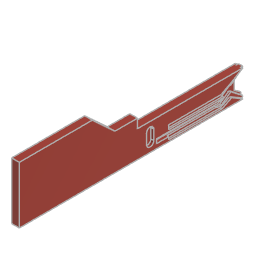
4ks (Autodesk Fusion 360 design; units mm, degrees)
Autodesk Fusion 360 part; units mm, degrees
note: some values were not read from the file. Set by a fixed rule: which face or edge a step refers to.
sketch "blade" plane through (0, 0, 0) normal (1, 0, 0) x (0, 1, 0)
  line L0 (0, 0) -> (0, 0.75) construction
  line L1 (0, 0.75) -> (25.25, 0.75)
  line L2 (25.25, 0.75) -> (25.25, 8.75)
  line L3 (25.25, 8.75) -> (0, 8.75)
  line L4 (0, 8.75) -> (0, 0.75)
  dimension "d13" = 0.75
  dimension "d14" = 25.25
  dimension "d15" = 8
  constraint coincident L0.start origin
  constraint vertical L0
  constraint horizontal L1
  constraint vertical L2
  constraint horizontal L3
  constraint vertical L4
  measures "d13" distance of L0.start L0.end
  measures "d14" distance of L0.end L1.end
  measures "d15" distance of L0.end L3.end
extrude "Extrude1" add sketch "blade" along normal blind 1.1 makes body 1
sketch "single track" plane through (1.1, 0, 0) normal (1, 0, 0) x (0, 1, 0)
  line L0 (0, 8.75) -> (0, 0.75)
  line L1 (0, 0.75) -> (25.25, 0.75)
  line L2 (25.25, 0.75) -> (25.25, 8.75)
  line L3 (25.25, 8.75) -> (0, 8.75)
  line L4 (0, 0.75) -> (0.9, 0.75) construction
  line L5 (0.9, 0.75) -> (4.4, 0.75) construction
  line L6 (4.4, 0.75) -> (7.9, 0.75) construction
  line L7 (7.9, 0.75) -> (11.4, 0.75) construction
  line L8 (11.4, 0.75) -> (14.9, 0.75) construction
  line L9 (14.9, 0.75) -> (18.4, 0.75) construction
  line L10 (18.4, 0.75) -> (21.9, 0.75) construction
  line L11 (21.9, 0.75) -> (21.9, 4.75) construction
  line L12 (21.9, 4.75) -> (25.25, 4.75)
  line L13 (0.9, 0.75) -> (0.9, 2.75) construction
  line L14 (4.4, 0.75) -> (4.4, 2.75) construction
  line L15 (7.9, 0.75) -> (7.9, 2.75) construction
  line L16 (11.4, 0.75) -> (11.4, 2.75) construction
  line L17 (14.9, 0.75) -> (14.9, 2.75) construction
  line L18 (18.4, 0.75) -> (18.4, 2.75) construction
  circle A0 centre (0.9, 2.75) radius 0.6 construction
  circle A1 centre (4.4, 2.75) radius 0.6 construction
  circle A2 centre (7.9, 2.75) radius 0.6 construction
  circle A3 centre (11.4, 2.75) radius 0.6 construction
  circle A4 centre (14.9, 2.75) radius 0.6 construction
  circle A5 centre (18.4, 2.75) radius 0.85 construction
  line L19 (0.9, 2.75) -> (0, 2.75)
  line L20 (0, 0.75) -> (0, 2.75) construction
  line L21 (0.9, 2.75) -> (1.2, 2.75)
  line L22 (4.4, 2.75) -> (4.1, 2.75)
  line L23 (4.4, 2.75) -> (4.7, 2.75)
  line L24 (7.9, 2.75) -> (7.6, 2.75)
  line L25 (7.9, 2.75) -> (8.2, 2.75)
  line L26 (11.4, 2.75) -> (11.1, 2.75)
  line L27 (11.4, 2.75) -> (11.7, 2.75)
  line L28 (14.9, 2.75) -> (14.6, 2.75)
  line L29 (14.9, 2.75) -> (15.2, 2.75)
  line L30 (18.4, 2.75) -> (18.1, 2.75)
  line L31 (18.4, 2.75) -> (18.7, 2.75)
  line L32 (21.9, 4.75) -> (21.6, 4.75)
  line L33 (1.2, 2.75) -> (4.1, 2.75)
  line L34 (4.7, 2.75) -> (7.6, 2.75)
  line L35 (8.2, 2.75) -> (11.1, 2.75)
  line L36 (11.7, 2.75) -> (14.6, 2.75)
  line L37 (15.2, 2.75) -> (18.1, 2.75)
  line L38 (18.7, 2.75) -> (21.6, 4.75)
  dimension "d18" = 0.9
  dimension "d19" = 3.5
  dimension "d20" = 3.5
  dimension "d21" = 3.5
  dimension "d22" = 3.5
  dimension "d23" = 3.5
  dimension "d24" = 3.5
  dimension "d25" = 2
  dimension "d26" = 2
  dimension "d27" = 2
  dimension "d28" = 2
  dimension "d29" = 2
  dimension "d30" = 2
  dimension "d31" = 1.2
  dimension "d32" = 1.2
  dimension "d33" = 1.2
  dimension "d34" = 1.2
  dimension "d35" = 1.2
  dimension "d36" = 1.7
  dimension "d37" = 0.3
  dimension "d38" = 0.3
  dimension "d39" = 0.3
  dimension "d40" = 0.3
  dimension "d41" = 0.3
  dimension "d42" = 0.3
  dimension "d43" = 0.3
  dimension "d44" = 0.3
  dimension "d45" = 0.3
  dimension "d46" = 0.3
  dimension "d47" = 0.3
  dimension "d48" = 0.3
  constraint coincident L0.end L1.start
  constraint coincident L1 L4.end
  constraint parallel L1 L5
  constraint parallel L1 L6
  constraint parallel L1 L7
  constraint parallel L1 L8
  constraint parallel L1 L9
  constraint parallel L1 L10
  constraint perpendicular L10 L11
  constraint midpoint L2 L12.end
  constraint perpendicular L2 L12
  constraint perpendicular L4 L13
  constraint perpendicular L5 L14
  constraint perpendicular L6 L15
  constraint perpendicular L8 L16
  constraint perpendicular L9 L17
  constraint perpendicular L10 L18
  constraint coincident L13.end A0.centre
  constraint coincident L14.end A1.centre
  constraint coincident L15.end A2.centre
  constraint coincident L16.end A3.centre
  constraint coincident L17.end A4.centre
  constraint coincident L18.end A5.centre
  constraint coincident L0 L19.end
  constraint perpendicular L0 L19
  constraint perpendicular L13 L21
  constraint perpendicular L14 L22
  constraint perpendicular L14 L23
  constraint perpendicular L15 L24
  constraint perpendicular L15 L25
  constraint perpendicular L16 L26
  constraint perpendicular L16 L27
  constraint perpendicular L17 L28
  constraint perpendicular L17 L29
  constraint perpendicular L18 L30
  constraint perpendicular L18 L31
  constraint perpendicular L11 L32
  measures "d18" distance of L0.end L4.end
  measures "d19" distance of L4.end L5.end
  measures "d20" distance of L5.end L6.end
  measures "d21" distance of L6.end L7.end
  measures "d22" distance of L7.end L8.end
  measures "d23" distance of L8.end L9.end
  measures "d24" distance of L9.end L10.end
  measures "d25" distance of L4.end L13.end
  measures "d26" distance of L5.end L14.end
  measures "d27" distance of L6.end L15.end
  measures "d28" distance of L7.end L16.end
  measures "d29" distance of L8.end L17.end
  measures "d30" distance of L9.end L18.end
  measures "d31" diameter of A0
  measures "d32" diameter of A1
  measures "d33" diameter of A2
  measures "d34" diameter of A3
  measures "d35" diameter of A4
  measures "d36" diameter of A5
  measures "d37" distance of L13.end L21.end
  measures "d38" distance of L14.end L22.end
  measures "d39" distance of L14.end L23.end
  measures "d40" distance of L15.end L24.end
  measures "d41" distance of L15.end L25.end
  measures "d42" distance of L16.end L26.end
  measures "d43" distance of L16.end L27.end
  measures "d44" distance of L17.end L28.end
  measures "d45" distance of L17.end L29.end
  measures "d46" distance of L18.end L30.end
  measures "d47" distance of L18.end L31.end
  measures "d48" distance of L11.end L32.end
sketch "single track cutter" plane through (0, 0, 0) normal (0, -1, 0) x (1, 0, 0)
  line L0 (0, 8.75) -> (0, 0.75)
  line L1 (0, 0.75) -> (1.1, 0.75)
  line L2 (1.1, 0.75) -> (1.1, 8.75)
  line L3 (1.1, 8.75) -> (0, 8.75)
  line L4 (1.1, 2.75) -> (1.1, 2.15)
  line L5 (1.1, 2.75) -> (1.1, 3.35)
  line L6 (1.1, 3.35) -> (0.1, 3.35)
  line L7 (0.1, 3.35) -> (0.1, 2.15)
  line L8 (0.1, 2.15) -> (1.1, 2.15)
  point P0 (1.1, 2.75)
  dimension "d49" = 0.6
  dimension "d50" = 0.6
  dimension "d51" = 1
  constraint vertical L4
  constraint coincident P0 L4.start
  constraint parallel L2 L5
  constraint perpendicular L5 L6
  constraint perpendicular L6 L7
  constraint perpendicular L4 L8
  measures "d49" distance of P0 L4.end
  measures "d50" distance of P0 L5.end
  measures "d51" distance of L5.end L6.end
sketch "wider single track" plane through (1.1, 0, 0) normal (1, 0, 0) x (0, 1, 0)
  line L0 (0, 8.75) -> (0, 0.75)
  line L1 (0, 0.75) -> (25.25, 0.75)
  line L2 (25.25, 0.75) -> (25.25, 8.75)
  line L3 (25.25, 8.75) -> (0, 8.75)
  line L4 (0, 0.75) -> (18.4, 0.75) construction
  line L5 (18.4, 0.75) -> (21.9, 0.75) construction
  line L6 (21.9, 0.75) -> (21.9, 4.75) construction
  line L7 (21.9, 4.75) -> (25.25, 4.75)
  line L8 (18.4, 0.75) -> (18.4, 2.75) construction
  line L9 (18.4, 2.75) -> (18.15, 2.5) construction
  line L10 (18.4, 2.75) -> (18.31, 2.75) construction
  line L11 (18.4, 2.75) -> (18.15, 3) construction
  line L12 (18.4, 2.75) -> (18.31, 2.75) construction
  line L13 (18.4, 2.75) -> (18.31, 2.75) construction
  line L14 (18.15, 3) -> (18.15, 3.6) construction
  line L15 (18.15, 2.5) -> (18.15, 1.9) construction
  line L16 (18.4, 2.75) -> (18.6954, 2.75) construction
  arc A0 (18.6954, 2.75) -> (18.15, 3.6) centre (18.15, 3) ccw
  arc A1 (18.15, 1.9) -> (18.6954, 2.75) centre (18.15, 2.5) ccw
  line L17 (18.4, 2.75) -> (17.6046, 2.75) construction
  arc A2 (18.15, 3.6) -> (17.6046, 2.75) centre (18.15, 3) ccw
  arc A3 (17.6046, 2.75) -> (18.15, 1.9) centre (18.15, 2.5) ccw
  line L18 (18.4, 2.75) -> (18.15, 2.75)
  line L19 (18.4, 2.75) -> (18.825, 2.75)
  line L20 (21.9, 4.75) -> (21.6, 4.75)
  line L21 (18.825, 2.75) -> (21.6, 4.75)
  dimension "d52" = 18.4
  dimension "d53" = 3.5
  dimension "d54" = 2
  dimension "d55" = 45
  dimension "d56" = 0.3536
  dimension "d57" = 45
  dimension "d58" = 0.3536
  dimension "d59" = 0.09
  dimension "d60" = 0.6
  dimension "d61" = 0.6
  dimension "d62" = 0.25
  dimension "d63" = 0.425
  dimension "d64" = 0.3
  constraint coincident L0.end L1.start
  constraint perpendicular L0 L4
  constraint parallel L1 L5
  constraint perpendicular L5 L6
  constraint midpoint L2 L7.end
  constraint perpendicular L2 L7
  constraint perpendicular L4 L8
  constraint horizontal L10
  constraint horizontal L12
  constraint perpendicular L8 L13
  constraint vertical L14
  constraint parallel L8 L15
  constraint perpendicular L8 L16
  constraint coincident L16 A0.start
  constraint coincident L11.end L14.start
  constraint coincident L16.end A0.start
  constraint coincident L9 L15.start
  constraint perpendicular L8 L17
  constraint coincident L17 A2.end
  constraint coincident L17.end A2.end
  constraint perpendicular L8 L18
  constraint perpendicular L8 L19
  constraint perpendicular L6 L20
  measures "d52" distance of L0.end L4.end
  measures "d53" distance of L4.end L5.end
  measures "d54" distance of L4.end L8.end
  measures "d55" angle of L9 L10
  measures "d56" distance of L8.end L9.end
  measures "d57" angle of L11 L12
  measures "d58" distance of L8.end L11.end
  measures "d59" distance of L8.end L10.end
  measures "d60" distance of L11.end L14.end
  measures "d61" distance of L9.end L15.end
  measures "d62" distance of L8.end L18.end
  measures "d63" distance of L8.end L19.end
  measures "d64" distance of L6.end L20.end
sketch "wider single track cutter" plane through (0, 25.25, 0) normal (0, 1, 0) x (-1, 0, 0)
  line L0 (0, 0.75) -> (0, 8.75)
  line L1 (0, 8.75) -> (-1.1, 8.75)
  line L2 (-1.1, 8.75) -> (-1.1, 0.75)
  line L3 (-1.1, 0.75) -> (0, 0.75)
  line L4 (-1.1, 4.75) -> (-1.1, 3.9)
  line L5 (-1.1, 4.75) -> (-1.1, 5.6)
  line L6 (-1.1, 3.9) -> (-0.1, 3.9)
  line L7 (-0.1, 3.9) -> (-0.1, 5.6)
  line L8 (-0.1, 5.6) -> (-1.1, 5.6)
  point P0 (-1.1, 4.75)
  dimension "d65" = 0.85
  dimension "d66" = 0.85
  dimension "d67" = 1
  constraint vertical L4
  constraint coincident P0 L4.start
  constraint parallel L2 L5
  constraint perpendicular L4 L6
  constraint perpendicular L6 L7
  constraint perpendicular L5 L8
  measures "d65" distance of P0 L4.end
  measures "d66" distance of P0 L5.end
  measures "d67" distance of L4.end L6.end
sketch "double track" plane through (1.1, 0, 0) normal (1, 0, 0) x (0, 1, 0)
  line L0 (0, 8.75) -> (0, 0.75)
  line L1 (0, 0.75) -> (25.25, 0.75)
  line L2 (25.25, 0.75) -> (25.25, 8.75)
  line L3 (25.25, 8.75) -> (0, 8.75)
  line L4 (0, 0.75) -> (3.5, 0.75) construction
  line L5 (3.5, 0.75) -> (4.4, 0.75) construction
  line L6 (4.4, 0.75) -> (7.9, 0.75) construction
  line L7 (7.9, 0.75) -> (11.4, 0.75) construction
  line L8 (11.4, 0.75) -> (14.9, 0.75) construction
  line L9 (14.9, 0.75) -> (18.4, 0.75) construction
  line L10 (18.4, 0.75) -> (21.9, 0.75) construction
  line L11 (21.9, 0.75) -> (21.9, 4.75) construction
  line L12 (21.9, 4.75) -> (25.25, 4.75) construction
  line L13 (3.5, 0.75) -> (3.5, 8.75) construction
  line L14 (4.4, 0.75) -> (4.4, 3.25) construction
  line L15 (7.9, 0.75) -> (7.9, 3.25) construction
  line L16 (11.4, 0.75) -> (11.4, 3.25) construction
  line L17 (14.9, 0.75) -> (14.9, 3.25) construction
  line L18 (18.4, 0.75) -> (18.4, 3.25) construction
  line L19 (4.4, 3.25) -> (4.4, 2) construction
  line L20 (4.4, 3.25) -> (4.4, 4.5) construction
  line L21 (7.9, 3.25) -> (7.9, 2) construction
  line L22 (7.9, 3.25) -> (7.9, 4.5) construction
  line L23 (11.4, 3.25) -> (11.4, 2) construction
  line L24 (11.4, 3.25) -> (11.4, 4.5) construction
  line L25 (14.9, 3.25) -> (14.9, 2) construction
  line L26 (14.9, 3.25) -> (14.9, 4.5) construction
  line L27 (18.4, 3.25) -> (18.4, 2) construction
  line L28 (18.4, 3.25) -> (18.4, 4.5) construction
  line L29 (21.9, 4.75) -> (21.9, 3.5) construction
  line L30 (21.9, 4.75) -> (21.9, 6) construction
  circle A0 centre (4.4, 2) radius 0.6 construction
  circle A1 centre (4.4, 4.5) radius 0.6 construction
  circle A2 centre (7.9, 2) radius 0.6 construction
  circle A3 centre (7.9, 4.5) radius 0.6 construction
  circle A4 centre (11.4, 2) radius 0.6 construction
  circle A5 centre (11.4, 4.5) radius 0.6 construction
  circle A6 centre (14.9, 2) radius 0.6 construction
  circle A7 centre (14.9, 4.5) radius 0.6 construction
  circle A8 centre (18.4, 2) radius 0.6 construction
  circle A9 centre (18.4, 4.5) radius 0.6 construction
  line L31 (4.4, 4.5) -> (3.5, 4.5)
  line L32 (4.4, 2) -> (3.5, 2)
  line L33 (4.4, 2) -> (4.7, 2)
  line L34 (7.9, 2) -> (7.6, 2)
  line L35 (7.9, 2) -> (8.2, 2)
  line L36 (11.4, 2) -> (11.1, 2)
  line L37 (11.4, 2) -> (11.7, 2)
  line L38 (14.9, 2) -> (14.6, 2)
  line L39 (14.9, 2) -> (15.2, 2)
  line L40 (18.4, 2) -> (18.1, 2)
  line L41 (18.4, 2) -> (18.7, 2)
  line L42 (21.9, 3.5) -> (21.6, 3.5) construction
  line L43 (21.9, 6) -> (21.6, 6) construction
  line L44 (4.4, 4.5) -> (4.7, 4.5)
  line L45 (7.9, 4.5) -> (7.6, 4.5)
  line L46 (7.9, 4.5) -> (8.2, 4.5)
  line L47 (11.4, 4.5) -> (11.1, 4.5)
  line L48 (11.4, 4.5) -> (11.7, 4.5)
  line L49 (14.9, 4.5) -> (14.6, 4.5)
  line L50 (14.9, 4.5) -> (15.2, 4.5)
  line L51 (18.4, 4.5) -> (18.1, 4.5)
  line L52 (18.4, 4.5) -> (18.7, 4.5)
  line L53 (4.7, 2) -> (7.6, 2)
  line L54 (8.2, 2) -> (11.1, 2)
  line L55 (11.7, 2) -> (14.6, 2)
  line L56 (15.2, 2) -> (18.1, 2)
  line L57 (18.7, 2) -> (21.6, 3.5)
  line L58 (4.7, 4.5) -> (7.6, 4.5)
  line L59 (8.2, 4.5) -> (11.1, 4.5)
  line L60 (11.7, 4.5) -> (14.6, 4.5)
  line L61 (15.2, 4.5) -> (18.1, 4.5)
  line L62 (18.7, 4.5) -> (21.6, 6)
  line L63 (21.6, 3.5) -> (25.25, 1.3414)
  line L64 (21.6, 3.5) -> (25.25, 3.5) construction
  line L65 (25.25, 1.3414) -> (26.2829, 0.7305)
  line L66 (21.6, 6) -> (25.25, 8.1586)
  line L67 (21.6, 6) -> (25.25, 6) construction
  line L68 (25.25, 8.1586) -> (26.2829, 8.7695)
  dimension "d68" = 3.5
  dimension "d69" = 0.9
  dimension "d70" = 3.5
  dimension "d71" = 3.5
  dimension "d72" = 3.5
  dimension "d73" = 3.5
  dimension "d74" = 3.5
  dimension "d75" = 2.5
  dimension "d76" = 2.5
  dimension "d77" = 2.5
  dimension "d78" = 2.5
  dimension "d79" = 2.5
  dimension "d80" = 1.25
  dimension "d81" = 1.25
  dimension "d82" = 1.25
  dimension "d83" = 1.25
  dimension "d84" = 1.25
  dimension "d85" = 1.25
  dimension "d86" = 1.25
  dimension "d87" = 1.25
  dimension "d88" = 1.25
  dimension "d89" = 1.25
  dimension "d90" = 1.25
  dimension "d91" = 1.25
  dimension "d92" = 1.2
  dimension "d93" = 1.2
  dimension "d94" = 1.2
  dimension "d95" = 1.2
  dimension "d96" = 1.2
  dimension "d97" = 1.2
  dimension "d98" = 1.2
  dimension "d99" = 1.2
  dimension "d100" = 1.2
  dimension "d101" = 1.2
  dimension "d102" = 0.3
  dimension "d103" = 0.3
  dimension "d104" = 0.3
  dimension "d105" = 0.3
  dimension "d106" = 0.3
  dimension "d107" = 0.3
  dimension "d108" = 0.3
  dimension "d109" = 0.3
  dimension "d110" = 0.3
  dimension "d111" = 0.3
  dimension "d112" = 0.3
  dimension "d113" = 0.3
  dimension "d114" = 0.3
  dimension "d115" = 0.3
  dimension "d116" = 0.3
  dimension "d117" = 0.3
  dimension "d118" = 0.3
  dimension "d119" = 0.3
  dimension "d120" = 0.3
  dimension "d121" = 0.3
  dimension "d122" = 149.4
  dimension "d123" = 1.2
  dimension "d124" = 149.4
  dimension "d125" = 1.2
  constraint coincident L0.end L1.start
  constraint perpendicular L0 L4
  constraint parallel L1 L5
  constraint parallel L1 L6
  constraint parallel L1 L7
  constraint parallel L1 L8
  constraint parallel L1 L9
  constraint parallel L1 L10
  constraint perpendicular L10 L11
  constraint midpoint L2 L12.end
  constraint perpendicular L2 L12
  constraint coincident L3 L13.end
  constraint perpendicular L3 L13
  constraint perpendicular L5 L14
  constraint perpendicular L7 L15
  constraint perpendicular L7 L16
  constraint perpendicular L8 L17
  constraint perpendicular L1 L18
  constraint parallel L14 L19
  constraint parallel L19 L20
  constraint parallel L15 L21
  constraint parallel L15 L22
  constraint parallel L16 L23
  constraint parallel L23 L24
  constraint parallel L17 L25
  constraint parallel L17 L26
  constraint parallel L18 L27
  constraint parallel L18 L28
  constraint perpendicular L12 L29
  constraint perpendicular L12 L30
  constraint coincident L19.end A0.centre
  constraint coincident L20.end A1.centre
  constraint coincident L21.end A2.centre
  constraint coincident L22.end A3.centre
  constraint coincident L23.end A4.centre
  constraint coincident L24.end A5.centre
  constraint coincident L25.end A6.centre
  constraint coincident L26.end A7.centre
  constraint coincident L27.end A8.centre
  constraint coincident L28.end A9.centre
  constraint coincident L13 L31.end
  constraint perpendicular L13 L31
  constraint coincident L13 L32.end
  constraint perpendicular L13 L32
  constraint perpendicular L19 L33
  constraint perpendicular L21 L34
  constraint perpendicular L15 L35
  constraint perpendicular L16 L36
  constraint perpendicular L16 L37
  constraint perpendicular L17 L38
  constraint perpendicular L25 L39
  constraint perpendicular L18 L40
  constraint perpendicular L27 L41
  constraint perpendicular L11 L42
  constraint perpendicular L30 L43
  constraint perpendicular L20 L44
  constraint perpendicular L22 L45
  constraint perpendicular L22 L46
  constraint perpendicular L24 L47
  constraint perpendicular L24 L48
  constraint perpendicular L26 L49
  constraint perpendicular L26 L50
  constraint perpendicular L28 L51
  constraint perpendicular L28 L52
  constraint horizontal L64
  constraint coincident L2 L63.end
  constraint coincident L2 L64.end
  constraint parallel L63 L65
  constraint horizontal L67
  constraint coincident L2 L66.end
  constraint coincident L2 L67.end
  constraint parallel L66 L68
  measures "d68" distance of L0.end L4.end
  measures "d69" distance of L4.end L5.end
  measures "d70" distance of L5.end L6.end
  measures "d71" distance of L6.end L7.end
  measures "d72" distance of L7.end L8.end
  measures "d73" distance of L8.end L9.end
  measures "d74" distance of L9.end L10.end
  measures "d75" distance of L5.end L14.end
  measures "d76" distance of L6.end L15.end
  measures "d77" distance of L7.end L16.end
  measures "d78" distance of L8.end L17.end
  measures "d79" distance of L9.end L18.end
  measures "d80" distance of L14.end L19.end
  measures "d81" distance of L14.end L20.end
  measures "d82" distance of L15.end L21.end
  measures "d83" distance of L15.end L22.end
  measures "d84" distance of L16.end L23.end
  measures "d85" distance of L16.end L24.end
  measures "d86" distance of L17.end L25.end
  measures "d87" distance of L17.end L26.end
  measures "d88" distance of L18.end L27.end
  measures "d89" distance of L18.end L28.end
  measures "d90" distance of L11.end L29.end
  measures "d91" distance of L11.end L30.end
  measures "d92" diameter of A0
  measures "d93" diameter of A1
  measures "d94" diameter of A2
  measures "d95" diameter of A3
  measures "d96" diameter of A4
  measures "d97" diameter of A5
  measures "d98" diameter of A6
  measures "d99" diameter of A7
  measures "d100" diameter of A8
  measures "d101" diameter of A9
  measures "d102" distance of L19.end L33.end
  measures "d103" distance of L21.end L34.end
  measures "d104" distance of L21.end L35.end
  measures "d105" distance of L23.end L36.end
  measures "d106" distance of L23.end L37.end
  measures "d107" distance of L25.end L38.end
  measures "d108" distance of L25.end L39.end
  measures "d109" distance of L27.end L40.end
  measures "d110" distance of L27.end L41.end
  measures "d111" distance of L29.end L42.end
  measures "d112" distance of L30.end L43.end
  measures "d113" distance of L20.end L44.end
  measures "d114" distance of L22.end L45.end
  measures "d115" distance of L22.end L46.end
  measures "d116" distance of L24.end L47.end
  measures "d117" distance of L24.end L48.end
  measures "d118" distance of L26.end L49.end
  measures "d119" distance of L26.end L50.end
  measures "d120" distance of L28.end L51.end
  measures "d121" distance of L28.end L52.end
  measures "d122" angle of L63 L64
  measures "d123" distance of L63.end L65.end
  measures "d124" angle of L66 L67
  measures "d125" distance of L66.end L68.end
ref_plane "WorkPlane1" through (0.55, 3.5, 4.75) normal (0, -1, 0) x (0, 0, -1)
sketch "double track cutter" plane through (0, 3.5, 0) normal (0, -1, 0) x (-1, 0, 0)
  line L0 (-1.1, -2) -> (-1.1, -1.4)
  line L1 (-1.1, -4.5) -> (-1.1, -3.9)
  line L2 (-1.1, -4.5) -> (-1.1, -5.1)
  line L3 (-1.1, -2) -> (-1.1, -2.6)
  line L4 (-1.1, -5.1) -> (-0.6, -5.1)
  line L5 (-1.1, -1.4) -> (-0.6, -1.4)
  line L6 (-0.6, -1.4) -> (-0.6, -2.6)
  line L7 (-0.6, -2.6) -> (-1.1, -2.6)
  line L8 (-0.6, -5.1) -> (-0.6, -3.9)
  line L9 (-0.6, -3.9) -> (-1.1, -3.9)
  point P0 (-1.1, -2)
  point P1 (-1.1, -4.5)
  dimension "d127" = 0.6
  dimension "d128" = 0.6
  dimension "d129" = 0.6
  dimension "d130" = 0.6
  dimension "d131" = 0.5
  dimension "d132" = 0.5
  constraint vertical L0
  constraint coincident P0 L0.start
  constraint vertical L1
  constraint coincident P1 L1.start
  constraint parallel L1 L2
  constraint parallel L0 L3
  constraint perpendicular L2 L4
  constraint perpendicular L0 L5
  constraint perpendicular L5 L6
  constraint perpendicular L3 L7
  constraint perpendicular L4 L8
  constraint perpendicular L1 L9
  measures "d127" distance of P0 L0.end
  measures "d128" distance of P1 L1.end
  measures "d129" distance of P1 L2.end
  measures "d130" distance of P0 L3.end
  measures "d131" distance of L2.end L4.end
  measures "d132" distance of L0.end L5.end
extrude "sidebar hole extension" add 1 faces at (0.3667, 0, 6.0833) along direction (0, -1, 0) blind 5.5 on bodies 1 bodies 1
sketch "sidebar hole" plane through (1.1, 0, 0) normal (1, 0, 0) x (0, 1, 0)
  line L0 (-5.5, 0.75) -> (25.25, 0.75)
  line L1 (25.25, 0.75) -> (25.25, 8.75)
  line L2 (25.25, 8.75) -> (-5.5, 8.75)
  line L3 (-5.5, 8.75) -> (-5.5, 0.75)
  line L4 (-5.5, 0.75) -> (0, 0.75) construction
  line L5 (0, 0.75) -> (0, 4.75) construction
  line L6 (0, 4.75) -> (-2.9, 4.75) construction
  line L7 (-2.9, 4.75) -> (-2.9, 3.3)
  line L8 (-2.9, 3.3) -> (-2.9, 2.25) construction
  line L9 (-2.9, 2.25) -> (-0.8, 2.25) construction
  line L10 (-2.9, 4.75) -> (-2.9, 6.2)
  line L11 (-2.9, 6.2) -> (-2.9, 7.25) construction
  line L12 (-2.9, 7.25) -> (-0.8, 7.25) construction
  line L13 (-0.8, 7.25) -> (-0.8, 6.2) construction
  line L14 (-0.8, 2.25) -> (-0.8, 3.3) construction
  line L15 (-0.8, 3.3) -> (-0.8, 6.2)
  arc A0 (-0.8, 6.2) -> (-2.9, 6.2) centre (-1.85, 6.2) ccw
  arc A1 (-2.9, 3.3) -> (-0.8, 3.3) centre (-1.85, 3.3) ccw
  dimension "d135" = 5.5
  dimension "d136" = 4
  dimension "d137" = 2.9
  dimension "d138" = 1.45
  dimension "d139" = 1.05
  dimension "d140" = 2.1
  dimension "d141" = 1.45
  dimension "d142" = 1.05
  dimension "d143" = 2.1
  dimension "d144" = 1.05
  dimension "d145" = 1.05
  constraint coincident L0.start L3.end
  constraint perpendicular L3 L4
  constraint perpendicular L4 L5
  constraint perpendicular L5 L6
  constraint perpendicular L6 L7
  constraint parallel L7 L8
  constraint perpendicular L8 L9
  constraint perpendicular L6 L10
  constraint parallel L10 L11
  constraint perpendicular L11 L12
  constraint perpendicular L12 L13
  constraint perpendicular L9 L14
  constraint tangent L12 A0
  constraint tangent L9 A1
  measures "d135" distance of L0.start L4.end
  measures "d136" distance of L4.end L5.end
  measures "d137" distance of L5.end L6.end
  measures "d138" distance of L6.end L7.end
  measures "d139" distance of L7.end L8.end
  measures "d140" distance of L8.end L9.end
  measures "d141" distance of L6.end L10.end
  measures "d142" distance of L10.end L11.end
  measures "d143" distance of L11.end L12.end
  measures "d144" distance of L12.end L13.end
  measures "d145" distance of L9.end L14.end
sketch "feed ramp" plane through (1.1, 0, 0) normal (1, 0, 0) x (0, 1, 0)
  line L0 (-5.5, 0.75) -> (25.25, 0.75)
  line L1 (25.25, 0.75) -> (25.25, 8.75)
  line L2 (25.25, 8.75) -> (-5.5, 8.75)
  line L3 (-5.5, 8.75) -> (-5.5, 0.75)
  line L4 (25.25, 0.75) -> (25.25, 4.75) construction
  line L5 (25.25, 4.75) -> (23.35, 4.75) construction
  line L6 (23.35, 4.75) -> (23.35, 6.25)
  line L7 (23.35, 4.75) -> (23.35, 3.25)
  line L8 (23.35, 3.25) -> (25.25, 1.9196)
  line L9 (23.35, 3.25) -> (25.25, 3.25) construction
  line L10 (23.35, 6.25) -> (25.25, 7.5804)
  line L11 (23.35, 6.25) -> (25.25, 6.25) construction
  line L12 (25.25, 1.9196) -> (25.25, 1.2696) construction
  line L13 (25.25, 7.5804) -> (25.25, 8.2304) construction
  line L14 (25.25, 8.2304) -> (20.7953, 4.75)
  line L15 (25.25, 8.2304) -> (26.15, 8.2304) construction
  line L16 (25.25, 1.2696) -> (20.7953, 4.75)
  line L17 (25.25, 1.2696) -> (26.15, 1.2696) construction
  line L18 (25.25, 1.2696) -> (26.15, 1.2696) construction
  line L19 (25.25, 8.2304) -> (26.15, 8.2304) construction
  dimension "d146" = 1.9
  dimension "d147" = 1.5
  dimension "d148" = 1.5
  dimension "d149" = 35
  dimension "d150" = 35
  dimension "d151" = 0.65
  dimension "d152" = 0.65
  dimension "d153" = 142
  dimension "d154" = 142
  dimension "d155" = 0.9
  dimension "d156" = 0.9
  constraint coincident L0.end L1.start
  constraint midpoint L1 L4.end
  constraint perpendicular L4 L5
  constraint perpendicular L5 L6
  constraint perpendicular L5 L7
  constraint horizontal L9
  constraint coincident L4 L8.end
  constraint coincident L4 L9.end
  constraint horizontal L11
  constraint coincident L1 L10.end
  constraint coincident L1 L11.end
  constraint parallel L4 L12
  constraint parallel L1 L13
  constraint horizontal L15
  constraint horizontal L17
  constraint coincident L14 L16.end
  constraint coincident L14.end L16.end
  constraint perpendicular L4 L18
  constraint perpendicular L13 L19
  measures "d146" distance of L4.end L5.end
  measures "d147" distance of L5.end L6.end
  measures "d148" distance of L5.end L7.end
  measures "d149" angle of L8 L9
  measures "d150" angle of L10 L11
  measures "d151" distance of L8.end L12.end
  measures "d152" distance of L10.end L13.end
  measures "d153" angle of L14 L15
  measures "d154" angle of L16 L17
  measures "d155" distance of L12.end L17.end
  measures "d156" distance of L13.end L15.end
sketch "bow" plane through (1.1, 0, 0) normal (1, 0, 0) x (0, 1, 0)
  line L0 (-5.5, 0.75) -> (25.25, 0.75)
  line L1 (25.25, 0.75) -> (25.25, 8.75)
  line L2 (25.25, 8.75) -> (-5.5, 8.75)
  line L3 (-5.5, 8.75) -> (-5.5, 0.75)
  line L4 (-5.5, 0.75) -> (-39.5, 0.75)
  line L5 (-39.5, 0.75) -> (-39.5, 17.25)
  line L6 (-5.5, 8.75) -> (-5.5, 11.25)
  line L7 (-5.5, 11.25) -> (-12, 11.25)
  line L8 (-39.5, 17.25) -> (-18.5, 17.25)
  line L9 (-18.5, 17.25) -> (-12, 11.25)
  dimension "d157" = 34
  dimension "d158" = 16.5
  dimension "d159" = 2.5
  dimension "d160" = 6.5
  dimension "d161" = 21
  constraint coincident L0.start L3.end
  constraint perpendicular L3 L4
  constraint perpendicular L4 L5
  constraint coincident L2.end L3.start
  constraint perpendicular L2 L6
  constraint perpendicular L6 L7
  constraint perpendicular L5 L8
  measures "d157" distance of L0.start L4.end
  measures "d158" distance of L4.end L5.end
  measures "d159" distance of L2.end L6.end
  measures "d160" distance of L6.end L7.end
  measures "d161" distance of L5.end L8.end
extrude "Extrude3" cut sketch "sidebar hole" against normal blind 0.85 contours L7 L10 L15 A0 A1 bodies 1
extrude "Extrude4" cut sketch "feed ramp" against normal blind 1.1 contours L1 L6 L7 L8 L10 bodies 1
extrude "Extrude5" cut sketch "feed ramp" against normal blind 1 contours L1 L6 L7 L8 L10 L14 L16 bodies 1
extrude "Extrude6" cut sketch "wider single track" against normal blind 1 contours A0 A1 A2 A3 bodies 1
sweep "Sweep1" cut profiles "wider single track cutter" path "wider single track" along L18 L19 L21 L20 L7 section 1 contours L2 L4 L5 L6 L7 L8 bodies 1
sweep "Sweep2" cut profiles "single track cutter" path "single track" along L12 L32 L38 L31 L30 L37 L29 L28 L36 L27 L26 L35 L25 L24 L34 L23 L22 L33 L21 L19 section 1 contours L2 L4 L5 L6 L7 L8 bodies 1
sweep "Sweep3" cut profiles "double track cutter" path "double track" along L65 L63 L57 L41 L40 L56 L39 L38 L55 L37 L36 L54 L35 L34 L53 L33 L32 section 1 contours L0 L3 L5 L6 L7 bodies 1
sweep "Sweep4" cut profiles "double track cutter" path "double track" along L68 L66 L62 L52 L51 L61 L50 L49 L60 L48 L47 L59 L46 L45 L58 L44 L31 section 1 contours L1 L2 L4 L8 L9 bodies 1
copy_body "CopyPasteBodies1" bodies 1 makes body 2
move_body "Move1" bodies 2 to x (-1, 0, 0) y (0, 1, 0) z (0, 0, -1) at (0, 0, 1.5)
move_body "Move2" bodies 2 to x (1, 0, 0) y (0, 1, 0) z (0, 0, 1) at (0, 0, 8)
extrude "Extrude7" add sketch "bow" against normal blind 2.2 contours L3 L4 L5 L6 L7 L8 L9 bodies 1 2
move_face "OffsetFaces1" offset -0.125 2 faces at (0.2, 4.6904, 8.75) (0.2, -17.9762, 0.75) on bodies 1
equation "Single1 = 1 mm"
equation "Single2 = 1 mm"
equation "Single3 = 1 mm"
equation "Single4 = 1 mm"
equation "Single5 = 1 mm"
equation "Single6 = 1 mm"
equation "Double1 = 1 mm"
equation "Double2 = 1 mm"
equation "Double3 = 1 mm"
equation "Double4 = 1 mm"
equation "Double5 = 1 mm"
equation "TrackToleranceAdd = 0 mm"
equation "d20 = d19"
equation "d21 = d19"
equation "d22 = d19"
equation "d23 = d19"
equation "d24 = d19"
equation "d25 = 1.5 mm + 0.5 * Single1"
equation "d26 = 1.5 mm + 0.5 * Single2"
equation "d27 = 1.5 mm + 0.5 * Single3"
equation "d28 = 1.5 mm + 0.5 * Single4"
equation "d29 = 1.5 mm + 0.5 * Single5"
equation "d30 = 1.5 mm + 0.5 * Single6"
equation "d31 = 1.2 mm + TrackToleranceAdd"
equation "d32 = d31"
equation "d33 = d31"
equation "d34 = d31"
equation "d35 = d31"
equation "d36 = 1.7 mm + TrackToleranceAdd"
equation "d37 = 0.3 mm + 0.5 * TrackToleranceAdd"
equation "d38 = d37"
equation "d39 = d37"
equation "d40 = d37"
equation "d41 = d37"
equation "d42 = d37"
equation "d43 = d37"
equation "d44 = d37"
equation "d45 = d37"
equation "d46 = d37"
equation "d47 = d37"
equation "d48 = d37"
equation "d49 = 0.5 * d31"
equation "d50 = d49"
equation "d52 = d18 + ( d19 * 5 )"
equation "d53 = d19"
equation "d54 = d30"
equation "d56 = 2 * ( 0.5 * ( d36 - d31 ) ) * sin(45 deg)"
equation "d57 = d55"
equation "d58 = d56"
equation "d59 = 0.1 * d18"
equation "d60 = 0.5 * d31"
equation "d61 = d60"
equation "d62 = 0.5 * ( d36 - d31 )"
equation "d63 = 0.25 * d36"
equation "d64 = d37"
equation "d65 = 0.5 * d36"
equation "d66 = d65"
equation "d67 = d51"
equation "d68 = d19"
equation "d69 = d18"
equation "d70 = d19"
equation "d71 = d19"
equation "d72 = d19"
equation "d73 = d19"
equation "d74 = d19"
equation "d75 = 2 mm + 0.5 * Double1"
equation "d76 = 2 mm + 0.5 * Double2"
equation "d77 = 2 mm + 0.5 * Double3"
equation "d78 = 2 mm + 0.5 * Double4"
equation "d79 = 2 mm + 0.5 * Double5"
equation "d81 = d80"
equation "d82 = d80"
equation "d83 = d80"
equation "d84 = d80"
equation "d85 = d80"
equation "d86 = d80"
equation "d87 = d80"
equation "d88 = d80"
equation "d89 = d80"
equation "d90 = d80"
equation "d91 = d80"
equation "d92 = d31"
equation "d93 = d31"
equation "d94 = d31"
equation "d95 = d31"
equation "d96 = d31"
equation "d97 = d31"
equation "d98 = d31"
equation "d99 = d31"
equation "d100 = d31"
equation "d101 = d31"
equation "d102 = d37"
equation "d103 = d37"
equation "d104 = d37"
equation "d105 = d37"
equation "d106 = d37"
equation "d107 = d37"
equation "d108 = d37"
equation "d109 = d37"
equation "d110 = d37"
equation "d111 = d37"
equation "d112 = d37"
equation "d113 = d37"
equation "d114 = d37"
equation "d115 = d37"
equation "d116 = d37"
equation "d117 = d37"
equation "d118 = d37"
equation "d119 = d37"
equation "d120 = d37"
equation "d121 = d37"
equation "d123 = d31"
equation "d124 = d122"
equation "d125 = d31"
equation "d127 = d50"
equation "d128 = d50"
equation "d129 = d50"
equation "d130 = d50"
equation "d131 = 0.5 * d51"
equation "d132 = d131"
equation "d139 = 2.5 mm - d138"
equation "d141 = d138"
equation "d142 = d139"
equation "d143 = d140"
equation "d144 = d139"
equation "d145 = d139"
equation "d148 = d147"
equation "d150 = d149"
equation "d152 = d151"
equation "d154 = d153"
equation "d155 = d18"
equation "d156 = d18"
equation "d166 = -d51"
equation "d168 = -d51"
named bodies: "blade", "blade (1)"
